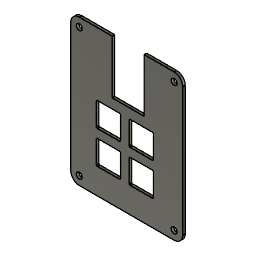
BluePrint top (Autodesk Fusion 360 design; units mm, degrees)
part number: 2025-12-15-16-17-42-386
Autodesk Fusion 360 part; units mm, degrees
sketch "plate-2025-12-11T20_48_07.428Z" plane through (0, 0, 0) normal (0, 1, 0) x (1, 0, 0)
sketch "plate-2025-12-11T20_48_07.428Z (1)" plane through (0, 0, 0) normal (0, 1, 0) x (1, 0, 0)
  line L0 (3.025, -2.525) -> (16.025, -2.525)
  line L1 (3.025, -16.525) -> (16.025, -16.525)
  line L2 (2.525, -3.025) -> (2.525, -16.025)
  line L3 (16.525, -3.025) -> (16.525, -16.025)
  arc A0 (3.025, -2.525) -> (2.525, -3.025) centre (3.025, -3.025) ccw
  arc A1 (16.525, -3.025) -> (16.025, -2.525) centre (16.025, -3.025) ccw
  arc A2 (2.525, -16.025) -> (3.025, -16.525) centre (3.025, -16.025) ccw
  arc A3 (16.025, -16.525) -> (16.525, -16.025) centre (16.025, -16.025) ccw
  line L4 (22.075, -2.525) -> (35.075, -2.525)
  line L5 (22.075, -16.525) -> (35.075, -16.525)
  line L6 (21.575, -3.025) -> (21.575, -16.025)
  line L7 (35.575, -3.025) -> (35.575, -16.025)
  arc A4 (22.075, -2.525) -> (21.575, -3.025) centre (22.075, -3.025) ccw
  arc A5 (35.575, -3.025) -> (35.075, -2.525) centre (35.075, -3.025) ccw
  arc A6 (21.575, -16.025) -> (22.075, -16.525) centre (22.075, -16.025) ccw
  arc A7 (35.075, -16.525) -> (35.575, -16.025) centre (35.075, -16.025) ccw
  line L8 (3.025, -21.575) -> (16.025, -21.575)
  line L9 (3.025, -35.575) -> (16.025, -35.575)
  line L10 (2.525, -22.075) -> (2.525, -35.075)
  line L11 (16.525, -22.075) -> (16.525, -35.075)
  arc A8 (3.025, -21.575) -> (2.525, -22.075) centre (3.025, -22.075) ccw
  arc A9 (16.525, -22.075) -> (16.025, -21.575) centre (16.025, -22.075) ccw
  arc A10 (2.525, -35.075) -> (3.025, -35.575) centre (3.025, -35.075) ccw
  arc A11 (16.025, -35.575) -> (16.525, -35.075) centre (16.025, -35.075) ccw
  line L12 (22.075, -21.575) -> (35.075, -21.575)
  line L13 (22.075, -35.575) -> (35.075, -35.575)
  line L14 (21.575, -22.075) -> (21.575, -35.075)
  line L15 (35.575, -22.075) -> (35.575, -35.075)
  arc A12 (22.075, -21.575) -> (21.575, -22.075) centre (22.075, -22.075) ccw
  arc A13 (35.575, -22.075) -> (35.075, -21.575) centre (35.075, -22.075) ccw
  arc A14 (21.575, -35.075) -> (22.075, -35.575) centre (22.075, -35.075) ccw
  arc A15 (35.075, -35.575) -> (35.575, -35.075) centre (35.075, -35.075) ccw
sketch "Sketch5" plane through (0, 0, 0) normal (0, 1, 0) x (1, 0, 0)
  line L0 (-12.375, -72.225) -> (52.625, -72.225)
  line L1 (52.625, -72.225) -> (52.625, 12.375)
  line L2 (52.625, 12.375) -> (-12.375, 12.375)
  line L3 (-12.375, 12.375) -> (-12.375, -72.225)
  line L4 (3.025, -2.525) -> (16.025, -2.525)
  line L5 (2.525, -3.025) -> (2.525, -16.025)
  line L6 (11.68, -72.225) -> (30.18, -72.225)
  line L7 (30.18, -72.225) -> (30.18, -41.225)
  line L8 (30.18, -41.225) -> (11.68, -41.225)
  line L9 (11.68, -41.225) -> (11.68, -72.225)
  circle A0 centre (-7.375, -67.225) radius 1.7
  circle A1 centre (47.625, -67.225) radius 1.7
  circle A2 centre (47.625, 7.375) radius 1.7
  circle A3 centre (-7.375, 7.375) radius 1.7
  dimension "d1" = 84.6
  dimension "d2" = 65
  dimension "d3" = 14.9
  dimension "d4" = 14.9
  dimension "d5" = 31
  dimension "d6" = 18.5
  dimension "d7" = 24.055
  dimension "d8" = 3.4
  dimension "d9" = 5
  dimension "d10" = 3.4
  dimension "d11" = 5
  dimension "d12" = 3.4
  dimension "d13" = 5
  dimension "d14" = 3.4
  dimension "d15" = 5
  dimension "d16" = 5
  dimension "d17" = 5
  dimension "d18" = 5
  dimension "d19" = 5
  constraint horizontal L0
  constraint vertical L1
  constraint horizontal L2
  constraint vertical L3
  constraint horizontal L6
  constraint vertical L7
  constraint horizontal L8
  constraint vertical L9
  constraint coincident L0 L6.start
  measures "d1" distance of L0.start L2.end
  measures "d2" distance of L0.start L0.end
  measures "d3" distance of L2 L4
  measures "d4" distance of L3 L5
  measures "d5" distance of L6.start L8.end
  measures "d6" distance of L7.end L8.end
  measures "d7" distance of L3 L9
  measures "d8" diameter of A0
  measures "d9" distance of L0 A0.centre
  measures "d10" diameter of A1
  measures "d11" distance of L1 A1.centre
  measures "d12" diameter of A2
  measures "d13" distance of L2 A2.centre
  measures "d14" diameter of A3
  measures "d15" distance of L2 A3.centre
  measures "d16" distance of L3 A3.centre
  measures "d17" distance of L1 A2.centre
  measures "d18" distance of L0 A1.centre
  measures "d19" distance of L3 A0.centre
extrude "Extrude1" add sketch "Sketch5" along normal blind 1.5 contours L0 L1 L2 L3 L7 L8 L9
extrude "Extrude2" cut sketch "plate-2025-12-11T20_48_07.428Z (1)" along normal through all
fillet "Fillet1" radius 5 4 edges at (-12.375, 0.75, 72.225) (52.625, 0.75, 72.225) (52.625, 0.75, -12.375) (-12.375, 0.75, -12.375)
